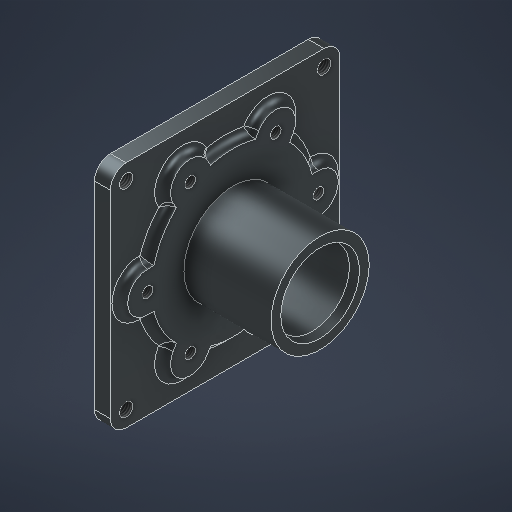
# Autodesk Inventor part: BASE COVER
Saved by Autodesk Inventor 2026.1 (Build 301233020, 233B)
## iProperties
Created: 2025-10-07
Part Number: BASE COVER
Material: Iron, Cast
Document SubType Name: Modeling
Designer: elaij
Density: 7.15 g/cm^3
Appearance: Iron Gray
Author: elaij
Autodesk Inventor part; units mm, degrees
ref_plane "YZ Plane" through (0, 0, 0) normal (1, 0, 0) x (0, 1, 0)
ref_plane "XZ Plane" through (0, 0, 0) normal (0, 1, 0) x (-1, 0, 0)
ref_plane "XY Plane" through (0, 0, 0) normal (0, 0, 1) x (1, 0, 0)
sketch "Sketch2" plane through (0, 0, 0) normal (1, 0, 0) x (0, 1, 0)
  line L0 (0, 0) -> (46.7654, -27)
  circle A0 centre (46.7654, -27) radius 12.5
  circle A1 centre (46.7654, 27) radius 12.5
  circle A2 centre (0, 54) radius 12.5
  circle A3 centre (-46.7654, 27) radius 12.5
  circle A4 centre (-46.7654, -27) radius 12.5
  circle A5 centre (0, -54) radius 12.5
  line L1 (0, 0) -> (12.8411, 0)
  arc A6 (49.3373, -14.7675) -> (49.3373, 14.7675) centre (0, 0) ccw
  arc A7 (51.7452, -15.4413) -> (51.7452, 15.4413) centre (0, 0) ccw
  arc A8 (11.8797, -50.1111) -> (37.4577, -35.3437) centre (0, 0) ccw
  arc A9 (-39.2452, -37.092) -> (-12.5, -52.5333) centre (0, 0) ccw
  arc A10 (-37.4577, -35.3437) -> (-11.8797, -50.1111) centre (0, 0) ccw
  arc A11 (-51.7452, 15.4413) -> (-51.7452, -15.4413) centre (0, 0) ccw
  arc A12 (-49.3373, 14.7675) -> (-49.3373, -14.7675) centre (0, 0) ccw
  arc A13 (37.4577, 35.3437) -> (11.8797, 50.1111) centre (0, 0) ccw
  arc A14 (-11.8797, 50.1111) -> (-37.4577, 35.3437) centre (0, 0) ccw
  arc A15 (39.2452, 37.092) -> (12.5, 52.5333) centre (0, 0) ccw
  arc A16 (-12.5, 52.5333) -> (-39.2452, 37.092) centre (0, 0) ccw
  line L2 (-40.5154, 37.8253) -> (53.0154, -16.1747)
  line L3 (-53.0154, 16.1747) -> (40.5154, -37.8253)
  line L4 (40.5154, 37.8253) -> (-53.0154, -16.1747)
  line L5 (-40.5154, -37.8253) -> (53.0154, 16.1747)
  line L6 (12.5, 54) -> (12.5, -54)
  line L7 (-12.5, 54) -> (-12.5, -54)
  arc A17 (12.5, -52.5333) -> (39.2452, -37.092) centre (0, 0) ccw
  arc A18 (39.3044, -37.0292) -> (46.7654, -27) centre (0, 0) ccw
  point P0 (12.5, 49.96)
  point P1 (-12.5, 49.96)
  point P2 (-37.0166, 35.8053)
  point P3 (-49.5166, 14.1547)
  point P4 (-49.5166, -14.1547)
  point P5 (-37.0166, -35.8053)
  point P6 (-12.5, -49.96)
  point P7 (12.5, -49.96)
  point P8 (49.5166, -14.1547)
  point P9 (37.0166, -35.8053)
  point P10 (49.5166, 14.1547)
  point P11 (37.0166, 35.8053)
  dimension "d11" = 360
  dimension "d13" = 30
  dimension "d15" = 25
  constraints: 51 point on circle, 19 centre point, 16 end point, 12 point on line, 12 tangent, 3 coincident, 1 horizontal, 13 other
  measures "d13" angle of L1 L0
  measures "d15" diameter of A0
extrude "Extrusion2" add sketch "Sketch2" against normal blind 5 contours L1 L6 L0 | L0 L5 L3 L7 L4 L2 L6 L1 | L5 L2 A6 A0 L0 | L6 L3 L5 | L6 L2 L5 | L0 A0 A8 L3 L6 | A0 A18 L0 | L0 A18 A0 | L5 L7 L3 | L3 L6 A8 A5 A10 L7 L5 | L5 A6 L2 | L2 L6 L4 A13 A1 A6 L5 | L3 A8 L6 | L2 L4 L6 | A6 L2 A0 | A0 L3 A8 | L7 L5 A10 A4 A12 L4 L3 | L3 L4 L7 | L7 A10 L5 | A6 A1 L5 | L6 A5 A8 | L4 L7 L2 | L2 L7 A14 A2 A13 L6 L4 | L6 A13 L4 | L4 A12 L3 | L3 A12 A3 A14 L2 L7 L4 | L5 A4 A10 | A10 A5 L7 | A1 | A5 | L2 A14 L7 | L4 A1 A13 | A13 A2 L6 | L3 A3 A12 | A12 A4 L4 | A4 | A14 A3 L2 | L7 A2 A14 | A2 | A3
sketch "Sketch5" plane through (-5, 0, 0) normal (-1, 0, 0) x (0, 0, 1)
  line L0 (-62.5, 62.5) -> (62.5, 62.5)
  line L1 (62.5, 62.5) -> (62.5, -62.5)
  line L2 (62.5, -62.5) -> (-62.5, -62.5)
  line L3 (-62.5, -62.5) -> (-62.5, 62.5)
  circle A0 centre (62.5, 62.5) radius 10
  circle A1 centre (62.5, -62.5) radius 10
  circle A2 centre (-62.5, 62.5) radius 10
  circle A3 centre (-62.5, -62.5) radius 10
  line L4 (-72.5, 72.5) -> (72.5, 72.5)
  line L5 (72.5, 72.5) -> (72.5, -72.5)
  line L6 (72.5, -72.5) -> (-72.5, -72.5)
  line L7 (-72.5, -72.5) -> (-72.5, 72.5)
  point P0 (0, 0)
  point P1 (62.5, 72.5)
  point P2 (-62.5, 72.5)
  point P3 (-72.5, 62.5)
  point P4 (-72.5, -62.5)
  point P5 (-62.5, -72.5)
  point P6 (62.5, -72.5)
  point P7 (72.5, -62.5)
  point P8 (72.5, 62.5)
  dimension "d40" = 125
  dimension "d41" = 62.5
  dimension "d42" = 125
  dimension "d43" = 62.5
  dimension "d46" = 125
  dimension "d49" = 125
  dimension "d52" = 20
  constraints: 16 end point, 4 centre point, 4 parallel, 4 tangent, 3 horizontal, 2 perpendicular, 1 coincident, 1 vertical, 6 other
  measures "d40" distance between parallel lines of L1 L3
  measures "d41" distance from line of point (0, 0) L1
  measures "d42" distance between parallel lines of L2 L0
  measures "d43" distance from line of point (0, 0) L2
  measures "d46" distance of A0.centre A1.centre
  measures "d49" distance of A0.centre A2.centre
  measures "d52" diameter of A0
extrude "Extrusion5" add sketch "Sketch5" along normal blind 10 contours L3 A2 L0 | L0 A2 L3 | A2 L4 A0 L0 | L0 A0 L1 A1 L2 A3 L3 A2 | L3 A3 L7 A2 | A0 L1 L0 | L0 L1 A0 | A3 L2 L3 | L3 L2 A3 | A0 L5 A1 L1 | L2 A1 L6 A3 | A1 L2 L1 | L1 L2 A1
sketch "Sketch6" plane through (-15, 0, 0) normal (-1, 0, 0) x (0, 0, 1)
  line L0 (-62.5, 62.5) -> (62.5, 62.5)
  line L1 (62.5, 62.5) -> (62.5, -62.5)
  line L2 (62.5, -62.5) -> (-62.5, -62.5)
  line L3 (-62.5, -62.5) -> (-62.5, 62.5)
  circle A0 centre (62.5, 62.5) radius 10
  circle A1 centre (62.5, -62.5) radius 10
  circle A2 centre (-62.5, 62.5) radius 10
  circle A3 centre (-62.5, -62.5) radius 10
  line L4 (-72.5, 72.5) -> (72.5, 72.5)
  line L5 (72.5, 72.5) -> (72.5, -72.5)
  line L6 (72.5, -72.5) -> (-72.5, -72.5)
  line L7 (-72.5, -72.5) -> (-72.5, 72.5)
  point P0 (0, 0)
  point P1 (0, 0)
  point P2 (91.0413, 95.2532)
  point P3 (-33.9587, 95.2532)
  point P4 (-43.9587, 85.2532)
  point P5 (-43.9587, -39.7468)
  point P6 (-33.9587, -49.7468)
  point P7 (91.0413, -49.7468)
  point P8 (101.0413, -39.7468)
  point P9 (101.0413, 85.2532)
  point P10 (-62.5, -52.5)
  point P11 (-52.5, -62.5)
  point P12 (52.5, -62.5)
  point P13 (62.5, -52.5)
  point P14 (62.5, 52.5)
  point P15 (52.5, 62.5)
  point P16 (-52.5, 62.5)
  point P17 (-62.5, 52.5)
  dimension "d59" = 125
  dimension "d60" = 62.5
  dimension "d61" = 125
  dimension "d62" = 62.5
  dimension "d63" = 125
  dimension "d64" = 125
  dimension "d65" = 20
  dimension "d66" = 0
  dimension "d67" = 0
  constraints: 16 end point, 4 centre point, 4 parallel, 4 tangent, 3 horizontal, 2 perpendicular, 1 coincident, 1 vertical, 6 other
  measures "d59" distance between parallel lines of L1 L3
  measures "d60" distance from line of point (0, 0) L1
  measures "d61" distance between parallel lines of L2 L0
  measures "d62" distance from line of point (0, 0) L2
  measures "d63" distance of A0.centre A1.centre
  measures "d64" distance of A0.centre A2.centre
  measures "d65" diameter of A0
  measures "d66" distance of point (0, 0) point (0, 0)
  measures "d67" distance of point (0, 0) point (0, 0)
extrude "Extrusion6" cut sketch "Sketch6" against normal blind 4 contours L0 A0 L1 A1 L2 A3 L3 A2
sketch "Sketch7" plane through (-11, 0, 0) normal (-1, 0, 0) x (0, 0, 1)
  circle A0 centre (0, 0) radius 37.5
  dimension "d70" = 75
  constraints: 1 centre point, 1 coincident
  measures "d70" diameter of A0
extrude "Extrusion7" add sketch "Sketch7" along normal blind 15
sketch "Sketch8" plane through (0, 0, 0) normal (1, 0, 0) x (0, 0, -1)
  circle A0 centre (0, 0) radius 31
  dimension "d73" = 62
  constraints: 1 centre point, 1 coincident
  measures "d73" diameter of A0
extrude "Extrusion8" add sketch "Sketch8" along normal blind 55
sketch "Sketch9" plane through (-26, 0, 0) normal (-1, 0, 0) x (0, 0, 1)
  point P0 (0, 0)
  point P1 (0, 0)
  constraints: 1 coincident
hole "Hole1" at (-26, 0, 0) direction (1, 0, 0) diameter 25 end through all
fillet "Fillet2" radius 5 12 edges at (-5, 57.5907, -33.25) (-5, 25.75, -44.6003) (-5, 0, -66.5) (-5, -25.75, -44.6003) (-5, -57.5907, -33.25) (-5, -51.5, 0) (-5, -57.5907, 33.25) (-5, -25.75, 44.6003) (-5, 0, 66.5) (-5, 25.75, 44.6003) (-5, 57.5907, 33.25) (-5, 51.5, 0)
sketch "Sketch10" plane through (0, 0, 0) normal (1, 0, 0) x (0, 0, -1)
  arc A0 (37.8253, 40.5154) -> (16.1747, 53.0154) centre (27, 46.7654) ccw projected
  circle A1 centre (0, 0) radius 54
  point P0 (-27, 46.7654)
  point P1 (-54, 0)
  point P2 (-27, -46.7654)
  point P3 (27, -46.7654)
  point P4 (54, 0)
  dimension "d86" = 360
  constraints: 2 coincident, 10 other
hole "Hole2" at (0, 46.7654, -27) at (0, 0, -54) at (0, -46.7654, -27) at (0, -46.7654, 27) at (0, 0, 54) at (0, 46.7654, 27) direction (-1, 0, 0) diameter 6.647 end through all thread size "M8x1.25" class "6H" standard "ISO Metric profile"
sketch "Sketch11" plane through (-5, 0, 0) normal (1, 0, 0) x (0, 0, -1)
  arc A0 (62.5, -72.5) -> (72.5, -62.5) centre (62.5, -62.5) ccw projected
  arc A1 (-62.5, 72.5) -> (-72.5, 62.5) centre (-62.5, 62.5) ccw projected
  line L0 (62.5, -62.5) -> (-62.5, -62.5)
  line L1 (-62.5, -62.5) -> (-62.5, 62.5)
  line L2 (-62.5, 62.5) -> (62.5, 62.5)
  line L3 (62.5, 62.5) -> (62.5, -62.5)
  point P0 (0, 0)
  constraints: 8 end point, 4 coincident, 2 parallel, 1 horizontal, 1 perpendicular
hole "Hole3" at (-5, -62.5, -62.5) at (-5, -62.5, 62.5) at (-5, 62.5, 62.5) at (-5, 62.5, -62.5) direction (-1, 0, 0) diameter 8.376 end through all thread size "M10x1.5" class "6H" standard "ISO Metric profile"
fillet "Fillet3" radius 4 8 edges at (-11, 0, -62.5) (-11, 55.4289, -55.4289) (-11, 62.5, 0) (-11, 55.4289, 55.4289) (-11, 0, 62.5) (-11, -55.4289, -55.4289) (-11, -62.5, 0) (-11, -55.4289, 55.4289)
fillet "Fillet4" radius 2 2 edges at (-26, 0, -37.5) (-11, 0, -37.5)
sketch "Sketch12" plane through (55, 0, 0) normal (1, 0, 0) x (0, 0, -1)
  circle A0 centre (0, 0) radius 23.5
  dimension "d104" = 47
  constraints: 1 centre point, 1 coincident
  measures "d104" diameter of A0
extrude "Extrusion9" cut sketch "Sketch12" against normal blind 43
chamfer "Chamfer1" distance 5 angle 15 1 edges at (55, 0, 23.5) measured on face at (54.5, 0, 23.5)
body "Solid2"
